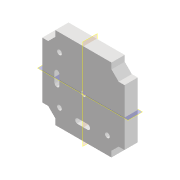
# Autodesk Inventor part: 20_Cube_Insert_Eyepiece
Saved by Autodesk Inventor 2022 (Build 260153000, 153)
## iProperties
Created: 2019-07-01
Part Number: 20_Cube_Insert_Eyepiece
Material: Generic
Document SubType Name: Modeling
Designer: diederichbenedict
Density: 1 g/cm^3
Appearance: Default
Author: diederichbenedict
Autodesk Inventor part; units mm, degrees
ref_plane "YZ Plane" through (0, 0, 0) normal (1, 0, 0) x (0, 1, 0)
ref_plane "XZ Plane" through (0, 0, 0) normal (0, 1, 0) x (-1, 0, 0)
ref_plane "Work Plane1" through (0, 0, 10) normal (0, 0, 1) x (1, 0, 0)
sketch "Sketch1" plane through (0, 0, 10) normal (0, 0, 1) x (1, 0, 0)
  line L0 (-4.0299, -0.3538) -> (-2.2322, 1.4439) construction
  arc A0 (-1.4439, 2.2322) -> (-2.2322, 1.4439) centre (-0.9299, 0.9299) ccw construction
  line L1 (-1.4439, 2.2322) -> (0.3538, 4.0299) construction
  line L2 (-37.8299, 42.8299) -> (-37.8299, 37.8299) construction
  line L3 (-37.8299, 37.8299) -> (-42.9208, 37.8299) construction
  line L4 (-37.8299, 42.2137) -> (-37.8299, 45.8299) construction
  line L5 (-37.8299, 45.8299) -> (-4.0299, 45.8299) construction
  line L6 (-4.0299, 45.8299) -> (-4.0299, 42.2137) construction
  line L7 (-4.0299, 4.0299) -> (0.3538, 4.0299) projected
  circle A1 centre (-20.9299, 20.9299) radius 17.5 projected
  line L8 (-20.9299, 58.9723) -> (17.1124, 20.9299) construction
  line L9 (17.1124, 20.9299) -> (-20.9299, -17.1124) construction
  line L10 (-20.9299, -17.1124) -> (-58.9723, 20.9299) construction
  line L11 (-58.9723, 20.9299) -> (-20.9299, 58.9723) construction
  line L12 (-20.9299, 58.9723) -> (-20.9299, -17.1124) construction
  line L13 (17.1124, 20.9299) -> (-58.9723, 20.9299) construction
  line L14 (-20.9299, 58.9723) -> (32.8701, 58.9723) construction
  line L15 (-43.4299, 43.4299) -> (1.5701, 43.4299) construction
  line L16 (1.5701, 43.4299) -> (1.5701, -1.5701) construction
  line L17 (1.5701, -1.5701) -> (-43.4299, -1.5701) construction
  line L18 (-43.4299, -1.5701) -> (-43.4299, 43.4299) construction
  line L19 (-43.4299, 43.4299) -> (1.5701, -1.5701) construction
  line L20 (1.5701, 43.4299) -> (-43.4299, -1.5701) construction
  line L21 (-43.4299, 5.3876) -> (-43.4299, 36.4723)
  line L22 (-43.4299, 36.4723) -> (-36.4723, 43.4299)
  line L23 (-36.4723, 43.4299) -> (-5.3876, 43.4299)
  line L24 (-5.3876, 43.4299) -> (1.5701, 36.4723)
  line L25 (1.5701, 36.4723) -> (1.5701, 5.3876)
  line L26 (1.5701, 5.3876) -> (-5.3876, -1.5701)
  line L27 (-5.3876, -1.5701) -> (-36.4723, -1.5701)
  line L28 (-36.4723, -1.5701) -> (-43.4299, 5.3876)
  line L29 (-4.0299, 42.2137) -> (-37.8299, 42.2137) projected
  line L30 (-4.0299, -0.3538) -> (-4.0299, 4.0299) projected
  circle A2 centre (-20.9299, 20.9299) radius 1.5
  line L31 (-10.9299, 10.9299) -> (-30.9299, 10.9299) construction
  line L32 (-30.9299, 10.9299) -> (-30.9299, 30.9299) construction
  line L33 (-30.9299, 30.9299) -> (-10.9299, 30.9299) construction
  line L34 (-10.9299, 30.9299) -> (-10.9299, 10.9299) construction
  line L35 (-10.9299, 10.9299) -> (-30.9299, 30.9299) construction
  line L36 (-30.9299, 10.9299) -> (-10.9299, 30.9299) construction
  circle A3 centre (-30.9299, 30.9299) radius 1.4
  circle A4 centre (-30.9299, 10.9299) radius 1.4
  circle A5 centre (-10.9299, 10.9299) radius 1.4
  line L37 (-45.8299, 37.8299) -> (-42.0723, 37.8299) construction
  line L38 (-42.1723, 37.7299) -> (-45.8299, 37.7299)
  line L39 (-45.8299, 37.7299) -> (-45.8299, 4.1299)
  line L40 (-45.8299, 4.1299) -> (-42.1723, 4.1299)
  line L41 (-42.1723, 4.1299) -> (-42.1723, 37.7299)
  line L42 (-45.8299, 4.0299) -> (-42.0723, 4.0299) construction
  line L43 (-45.8299, 37.8299) -> (-42.0723, 37.8299) projected
  line L44 (-37.7299, 45.8299) -> (-4.1299, 45.8299)
  line L45 (-4.1299, 45.8299) -> (-4.1299, 42.1723)
  line L46 (-4.1299, 42.1723) -> (-37.7299, 42.1723)
  line L47 (-37.7299, 42.1723) -> (-37.7299, 45.8299)
  line L48 (0.4701, 37.8299) -> (0.4701, 4.0299) construction
  line L49 (0.4701, 4.0299) -> (3.9701, 4.0299) construction
  line L50 (3.9701, 37.8299) -> (3.9701, 4.0299) construction
  line L51 (0.4701, 37.8299) -> (3.9701, 37.8299) construction
  line L52 (-45.8299, -3.9701) -> (-4.0299, -3.9701) construction
  line L53 (0.3124, 37.7299) -> (3.9701, 37.7299)
  line L54 (3.9701, 37.7299) -> (3.9701, 4.1299)
  line L55 (3.9701, 4.1299) -> (0.3124, 4.1299)
  line L56 (0.3124, 4.1299) -> (0.3124, 37.7299)
  line L57 (-4.1713, -0.3538) -> (-37.7299, -0.3538)
  line L58 (-37.7299, -0.3538) -> (-37.7299, -3.9701)
  line L59 (-37.7299, -3.9701) -> (-4.1713, -3.9701)
  line L60 (-4.1713, -3.9701) -> (-4.1713, -0.3538)
  point P0 (-37.8299, 4.0299)
  dimension "d18" = 53.8
  dimension "d19" = 45
  dimension "d20" = 53.8
  dimension "d21" = 45
  dimension "d22" = 45
  dimension "d30" = 20
  dimension "d31" = 20
  dimension "d32" = 2.8
  dimension "d33" = 2.8
  dimension "d34" = 2.8
  dimension "d35" = 3
  dimension "d36" = 0.1
  dimension "d37" = 0.1
  dimension "d38" = 0.1
  dimension "d39" = 0.1
  constraints: 86 end point, 21 point on line, 14 parallel, 8 perpendicular, 7 horizontal, 7 midpoint, 4 centre point, 4 coincident, 1 equal length
  measures "d18" distance of L8.start L8.end
  measures "d19" angle of L8 L14
  measures "d20" distance of L8.end L9.end
  measures "d21" distance of L16.end L17.end
  measures "d22" distance of L15.end L16.end
  measures "d30" distance of L32.end L33.end
  measures "d31" distance of L31.end L32.end
  measures "d32" diameter of A3
  measures "d33" diameter of A4
  measures "d34" diameter of A5
  measures "d35" diameter of A2
  measures "d36" distance between parallel lines of L38 L43
  measures "d37" distance between parallel lines of L40 L42
  measures "d38" distance between parallel lines of L45 L6
  measures "d39" distance between parallel lines of L4 L47
extrude "Extrusion1" add sketch "Sketch1" along normal blind 10 contours L30 L26 L57 L28 L41 L22 L46 L24 L56 L7 | L7 L26 L30 | L56 L24 L25 L26 | L26 L25 L24 L53 L54 L55 | L60 L59 L58 L57 L28 L27 L26 | L26 L27 L28 L57 | L46 L22 L29 L24 | L24 L29 L45 | L40 L39 L38 L22 L21 L28 | L28 L21 L22 L41 | L29 L22 L23 L24 | L24 L23 L22 L29 L47 L44 L45 | L47 L29 L22 | A1 | A2 | A3 | A4 | A5
sketch "Skizze4" plane through (0, 0, 20) normal (0, 0, 1) x (1, 0, 0)
  line L0 (-37.7299, 42.1723) -> (-42.1723, 37.7299) projected
  line L1 (-42.1723, 37.7299) -> (-45.8299, 37.7299) projected
  line L2 (-45.8299, 37.7299) -> (-45.8299, 4.1299) construction
  line L3 (-45.8299, 4.1299) -> (-42.1723, 4.1299) projected
  line L4 (-42.1723, 4.1299) -> (-37.6885, -0.3538) projected
  line L5 (-37.6885, -0.3538) -> (-37.7299, -0.3538) projected
  line L6 (-37.7299, -0.3538) -> (-37.7299, -3.9701) projected
  line L7 (-37.7299, -3.9701) -> (-4.1713, -3.9701) construction
  line L8 (-4.1713, -3.9701) -> (-4.1713, -0.3538) projected
  line L9 (-4.1713, -0.3538) -> (0.3124, 4.1299) projected
  line L10 (0.3124, 4.1299) -> (3.9701, 4.1299) projected
  line L11 (3.9701, 4.1299) -> (3.9701, 37.7299) construction
  line L12 (3.9701, 37.7299) -> (0.3124, 37.7299) projected
  line L13 (0.3124, 37.7299) -> (-4.1299, 42.1723) projected
  line L14 (-4.1299, 42.1723) -> (-4.1299, 45.8299) projected
  line L15 (-4.1299, 45.8299) -> (-37.7299, 45.8299) construction
  line L16 (-37.7299, 45.8299) -> (-37.7299, 42.1723) projected
  line L17 (-37.9299, 46.0299) -> (-3.9299, 46.0299) construction
  line L18 (-3.9299, 46.0299) -> (-3.9299, 42.2551)
  line L19 (-3.9299, 42.2551) -> (0.3953, 37.9299)
  line L20 (0.3953, 37.9299) -> (4.1701, 37.9299)
  line L21 (4.1701, 37.9299) -> (4.1701, 3.9299) construction
  line L22 (4.1701, 3.9299) -> (0.3953, 3.9299)
  line L23 (0.3953, 3.9299) -> (-3.9713, -0.4367)
  line L24 (-3.9713, -0.4367) -> (-3.9713, -4.1701)
  line L25 (-3.9713, -4.1701) -> (-37.9299, -4.1701) construction
  line L26 (-37.9299, -4.1701) -> (-37.9299, -0.3953)
  line L27 (-37.9299, -0.3953) -> (-42.2551, 3.9299)
  line L28 (-42.2551, 3.9299) -> (-46.0299, 3.9299)
  line L29 (-46.0299, 3.9299) -> (-46.0299, 37.9299) construction
  line L30 (-46.0299, 37.9299) -> (-42.2551, 37.9299)
  line L31 (-42.2551, 37.9299) -> (-37.9299, 42.2551)
  line L32 (-37.9299, 42.2551) -> (-37.9299, 46.0299)
  line L33 (-45.8299, 37.7299) -> (-45.8299, 37.9299)
  line L34 (-4.1299, 45.8299) -> (-37.7299, 45.8299) projected
  line L35 (-37.7299, 45.8299) -> (-37.9299, 45.8299)
  line L36 (-4.1299, 45.8299) -> (-3.9299, 45.8299)
  line L37 (3.9701, 37.7299) -> (3.9701, 37.9299)
  line L38 (3.9701, 4.1299) -> (3.9701, 37.7299) projected
  line L39 (3.9701, 4.1299) -> (3.9701, 3.9299)
  line L40 (-4.1713, -3.9701) -> (-3.9713, -3.9701)
  line L41 (-37.7299, -3.9701) -> (-37.9299, -3.9701)
  line L42 (-45.8299, 4.1299) -> (-45.8299, 3.9299)
  point P0 (0, 0)
  dimension "d40" = 0.2
  constraints: 48 end point, 12 point on line, 4 perpendicular, 15 other
  measures "d40" distance between parallel lines of L15 L17
extrude "IM_offset" add sketch "Skizze4" against normal up to surface (10 mm away)
ref_plane "Work Plane5" through (-37.9299, 20.9299, 10) normal (0, -1, 0) x (1, 0, 0)
ref_plane "Work Plane6" through (-20.9299, 3.9299, 10) normal (1, 0, 0) x (0, 0, -1)
sketch "Sketch24" plane through (0, 0, 10) normal (0, 0, -1) x (-1, 0, 0)
  line L0 (6.4299, 6.4299) -> (35.4299, 6.4299) construction
  line L1 (35.4299, 6.4299) -> (35.4299, 35.4299) construction
  line L2 (35.4299, 35.4299) -> (6.4299, 35.4299) construction
  line L3 (6.4299, 35.4299) -> (6.4299, 6.4299) construction
  line L4 (6.4299, 6.4299) -> (35.4299, 35.4299) construction
  line L5 (35.4299, 6.4299) -> (6.4299, 35.4299) construction
  point P0 (0, 0)
  point P1 (20.9299, 20.9299)
  dimension "d143" = 29
  dimension "d144" = 29
  constraints: 12 end point, 2 midpoint, 2 parallel, 1 horizontal, 1 perpendicular
  measures "d143" distance of L2.end L1.end
  measures "d144" distance of L1.end L0.end
hole "Hole1" at (-20.9299, 20.9299, 10) at (-6.4299, 6.4299, 10) at (-35.4299, 6.4299, 10) at (-35.4299, 35.4299, 10) direction (0, 0, 1) diameter 2.9 end through all counterbore diameter 6.5 counterbore depth 4
sketch "Sketch25" plane through (0, 0, 10) normal (0, 0, -1) x (-1, 0, 0)
  circle A0 centre (35.4299, 6.4299) radius 3.25 projected
  circle A1 centre (20.9299, 20.9299) radius 3.25 projected
  circle A2 centre (6.4299, 6.4299) radius 3.25 projected
  circle A3 centre (35.4299, 35.4299) radius 3.25 projected
  line L0 (3.9713, -3.9701) -> (37.9299, -3.9701) projected
  line L1 (37.9299, -3.9701) -> (37.9299, -0.3953) projected
  line L2 (37.9299, -0.3953) -> (42.2551, 3.9299) projected
  line L3 (42.2551, 3.9299) -> (45.8299, 3.9299) projected
  line L4 (45.8299, 3.9299) -> (45.8299, 37.9299) projected
  line L5 (45.8299, 37.9299) -> (42.2551, 37.9299) projected
  line L6 (42.2551, 37.9299) -> (37.9299, 42.2551) projected
  line L7 (37.9299, 42.2551) -> (37.9299, 45.8299) projected
  line L8 (37.9299, 45.8299) -> (3.9299, 45.8299) projected
  line L9 (3.9299, 45.8299) -> (3.9299, 42.2551) projected
  line L10 (3.9299, 42.2551) -> (-0.3953, 37.9299) projected
  line L11 (-0.3953, 37.9299) -> (-3.9701, 37.9299) projected
  line L12 (-3.9701, 37.9299) -> (-3.9701, 3.9299) projected
  line L13 (-3.9701, 3.9299) -> (-0.3953, 3.9299) projected
  line L14 (-0.3953, 3.9299) -> (3.9713, -0.4367) projected
  line L15 (3.9713, -0.4367) -> (3.9713, -3.9701) projected
  line L16 (36.9299, 17.9299) -> (36.9299, 23.9299) construction
  line L17 (38.4299, 17.9299) -> (38.4299, 23.9299)
  line L18 (35.4299, 23.9299) -> (35.4299, 17.9299)
  arc A4 (35.4299, 17.9299) -> (38.4299, 17.9299) centre (36.9299, 17.9299) ccw
  arc A5 (38.4299, 23.9299) -> (35.4299, 23.9299) centre (36.9299, 23.9299) ccw
  line L19 (18.4299, 4.8499) -> (24.4299, 4.8499) construction
  line L20 (18.4299, 3.3499) -> (24.4299, 3.3499)
  line L21 (24.4299, 6.3499) -> (18.4299, 6.3499)
  arc A6 (18.4299, 6.3499) -> (18.4299, 3.3499) centre (18.4299, 4.8499) ccw
  arc A7 (24.4299, 3.3499) -> (24.4299, 6.3499) centre (24.4299, 4.8499) ccw
  point P0 (0, 0)
  point P1 (36.9299, 20.9299)
  point P2 (21.4299, 4.8499)
  dimension "d152" = 3
  dimension "d153" = 3
  dimension "d154" = 3
  dimension "d155" = 3
  dimension "d164" = 1.58
  dimension "d165" = 1.5
  constraints: 16 end point, 8 point on circle, 8 tangent, 4 centre point, 2 midpoint, 2 parallel, 1 perpendicular, 1 vertical
  measures "d152" distance of point (36.93, 20.93) L16.end
  measures "d153" diameter of A5
  measures "d154" distance of point (21.43, 4.85) L19.end
  measures "d155" diameter of A7
  measures "d164" vertical distance of point (21.43, 4.85) A0.centre
  measures "d165" horizontal distance of point (36.93, 20.93) A0.centre
extrude "Extrusion20" cut sketch "Sketch25" against normal blind 10 contours A4 L18 A5 L17 | A6 L21 A7 L20
sketch "Sketch26" plane through (-45.8299, 3.9299, 10) normal (-1, 0, 0) x (0, 0, 1)
  line L0 (0, 14) -> (0, 20) projected
  line L1 (0, 20) -> (0, 14) projected
  circle A0 centre (5, 16.752) radius 1.45
  line L2 (10, 34) -> (10, 0) projected
  line L3 (0, 0) -> (0, 34) projected
  point P0 (-10, -3.9299)
  dimension "d158" = 2.9
  dimension "d172" = 5
  constraints: 1 centre point
  measures "d158" diameter of A0
  measures "d172" distance from line of L2 A0.centre
extrude "Extrusion21" cut sketch "Sketch26" against normal up to surface round surface about axis through (-20.9299, 20.9299, 12) along (0, 0, -1) radius 3.25 far side no
chamfer "Chamfer1" distance 0.5 angle 45 3 edges at (-35.4299, 33.9799, 14) (-35.4299, 4.9799, 14) (-6.4299, 4.9799, 14)
pattern_circular "Circular Pattern1" count 2 over 90 about axis through (-20.9299, 20.9299, 81.1342) along (0, 0, 1) of "Extrusion21"
body "Solid1"
